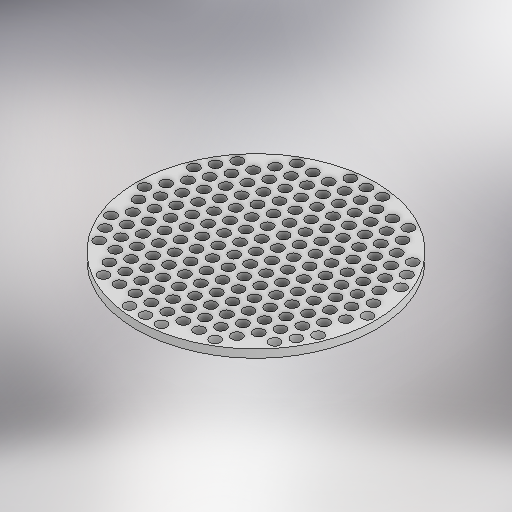
# Autodesk Inventor part: 滤网
Saved by Autodesk Inventor 2025 (Build 290162000, 162)
## iProperties
Created: 2025-03-16
Part Number: 滤网
Material: 常规
Document SubType Name: Modeling
Designer: ASUS
Density: 1 g/cm^3
Appearance: 默认
Author: ASUS
Autodesk Inventor part; units mm, degrees
ref_plane "YZ Plane" through (0, 0, 0) normal (1, 0, 0) x (0, 1, 0)
ref_plane "XZ Plane" through (0, 0, 0) normal (0, 1, 0) x (-1, 0, 0)
ref_plane "XY Plane" through (0, 0, 0) normal (0, 0, 1) x (1, 0, 0)
sketch "草图2" plane through (0, 0, 0) normal (0, 1, 0) x (1, 0, 0)
  circle A0 centre (0, 0) radius 1
  circle A1 centre (-1.5, -2.5981) radius 1
  circle A2 centre (1.5, -2.5981) radius 1
  circle A3 centre (-3, -20.7846) radius 1
  circle A4 centre (0, -20.7846) radius 1
  circle A5 centre (3, -20.7846) radius 1
  circle A6 centre (7.5, -18.1865) radius 1
  circle A7 centre (4.5, -18.1865) radius 1
  circle A8 centre (1.5, -18.1865) radius 1
  circle A9 centre (-1.5, -18.1865) radius 1
  circle A10 centre (-4.5, -18.1865) radius 1
  circle A11 centre (-7.5, -18.1865) radius 1
  circle A12 centre (-10.5, -18.1865) radius 1
  circle A13 centre (10.5, -18.1865) radius 1
  circle A14 centre (12, -15.5885) radius 1
  circle A15 centre (9, -15.5885) radius 1
  circle A16 centre (6, -15.5885) radius 1
  circle A17 centre (3, -15.5885) radius 1
  circle A18 centre (0, -15.5885) radius 1
  circle A19 centre (-3, -15.5885) radius 1
  circle A20 centre (-6, -15.5885) radius 1
  circle A21 centre (-9, -15.5885) radius 1
  circle A22 centre (-16.5, -12.9904) radius 1
  circle A23 centre (-13.5, -12.9904) radius 1
  circle A24 centre (-10.5, -12.9904) radius 1
  circle A25 centre (-7.5, -12.9904) radius 1
  circle A26 centre (-4.5, -12.9904) radius 1
  circle A27 centre (-1.5, -12.9904) radius 1
  circle A28 centre (1.5, -12.9904) radius 1
  circle A29 centre (4.5, -12.9904) radius 1
  circle A30 centre (7.5, -12.9904) radius 1
  circle A31 centre (10.5, -12.9904) radius 1
  circle A32 centre (13.5, -12.9904) radius 1
  circle A33 centre (16.5, -12.9904) radius 1
  circle A34 centre (18, -10.3923) radius 1
  circle A35 centre (15, -10.3923) radius 1
  circle A36 centre (12, -10.3923) radius 1
  circle A37 centre (9, -10.3923) radius 1
  circle A38 centre (6, -10.3923) radius 1
  circle A39 centre (3, -10.3923) radius 1
  circle A40 centre (0, -10.3923) radius 1
  circle A41 centre (-3, -10.3923) radius 1
  circle A42 centre (-6, -10.3923) radius 1
  circle A43 centre (-9, -10.3923) radius 1
  circle A44 centre (-12, -10.3923) radius 1
  circle A45 centre (-15, -10.3923) radius 1
  circle A46 centre (-18, -10.3923) radius 1
  circle A47 centre (-16.5, -7.7942) radius 1
  circle A48 centre (-13.5, -7.7942) radius 1
  circle A49 centre (-15, -5.1962) radius 1
  circle A50 centre (-18, -5.1962) radius 1
  circle A51 centre (-10.5, -7.7942) radius 1
  circle A52 centre (-7.5, -7.7942) radius 1
  circle A53 centre (-12, -5.1962) radius 1
  circle A54 centre (-6, -5.1962) radius 1
  circle A55 centre (-3, -5.1962) radius 1
  circle A56 centre (-4.5, -7.7942) radius 1
  circle A57 centre (-1.5, -7.7942) radius 1
  circle A58 centre (0, -5.1962) radius 1
  circle A59 centre (3, -5.1962) radius 1
  circle A60 centre (1.5, -7.7942) radius 1
  circle A61 centre (4.5, -7.7942) radius 1
  circle A62 centre (6, -5.1962) radius 1
  circle A63 centre (9, -5.1962) radius 1
  circle A64 centre (7.5, -7.7942) radius 1
  circle A65 centre (10.5, -7.7942) radius 1
  circle A66 centre (13.5, -7.7942) radius 1
  circle A67 centre (12, -5.1962) radius 1
  circle A68 centre (15, -5.1962) radius 1
  circle A69 centre (18, -5.1962) radius 1
  circle A70 centre (19.5, -7.7942) radius 1
  circle A71 centre (16.5, -7.7942) radius 1
  circle A72 centre (-12, -15.5885) radius 1
  circle A73 centre (-9, -5.1962) radius 1
  circle A74 centre (-19.5, -7.7942) radius 1
  circle A75 centre (-19.5, -2.5981) radius 1
  circle A76 centre (-16.5, -2.5981) radius 1
  circle A77 centre (-13.5, -2.5981) radius 1
  circle A78 centre (-10.5, -2.5981) radius 1
  circle A79 centre (-7.5, -2.5981) radius 1
  circle A80 centre (-4.5, -2.5981) radius 1
  circle A81 centre (4.5, -2.5981) radius 1
  circle A82 centre (7.5, -2.5981) radius 1
  circle A83 centre (10.5, -2.5981) radius 1
  circle A84 centre (13.5, -2.5981) radius 1
  circle A85 centre (16.5, -2.5981) radius 1
  circle A86 centre (19.5, -2.5981) radius 1
  line L0 (-23.4041, 0) -> (24.2926, 0) construction
  circle A87 centre (-1.5, 2.5981) radius 1
  circle A88 centre (1.5, 2.5981) radius 1
  circle A89 centre (-3, 20.7846) radius 1
  circle A90 centre (0, 20.7846) radius 1
  circle A91 centre (3, 20.7846) radius 1
  circle A92 centre (7.5, 18.1865) radius 1
  circle A93 centre (4.5, 18.1865) radius 1
  circle A94 centre (1.5, 18.1865) radius 1
  circle A95 centre (-1.5, 18.1865) radius 1
  circle A96 centre (-4.5, 18.1865) radius 1
  circle A97 centre (-7.5, 18.1865) radius 1
  circle A98 centre (-10.5, 18.1865) radius 1
  circle A99 centre (10.5, 18.1865) radius 1
  circle A100 centre (12, 15.5885) radius 1
  circle A101 centre (9, 15.5885) radius 1
  circle A102 centre (6, 15.5885) radius 1
  circle A103 centre (3, 15.5885) radius 1
  circle A104 centre (0, 15.5885) radius 1
  circle A105 centre (-3, 15.5885) radius 1
  circle A106 centre (-6, 15.5885) radius 1
  circle A107 centre (-9, 15.5885) radius 1
  circle A108 centre (-16.5, 12.9904) radius 1
  circle A109 centre (-13.5, 12.9904) radius 1
  circle A110 centre (-10.5, 12.9904) radius 1
  circle A111 centre (-7.5, 12.9904) radius 1
  circle A112 centre (-4.5, 12.9904) radius 1
  circle A113 centre (-1.5, 12.9904) radius 1
  circle A114 centre (1.5, 12.9904) radius 1
  circle A115 centre (4.5, 12.9904) radius 1
  circle A116 centre (7.5, 12.9904) radius 1
  circle A117 centre (10.5, 12.9904) radius 1
  circle A118 centre (13.5, 12.9904) radius 1
  circle A119 centre (16.5, 12.9904) radius 1
  circle A120 centre (18, 10.3923) radius 1
  circle A121 centre (15, 10.3923) radius 1
  circle A122 centre (12, 10.3923) radius 1
  circle A123 centre (9, 10.3923) radius 1
  circle A124 centre (6, 10.3923) radius 1
  circle A125 centre (3, 10.3923) radius 1
  circle A126 centre (0, 10.3923) radius 1
  circle A127 centre (-3, 10.3923) radius 1
  circle A128 centre (-6, 10.3923) radius 1
  circle A129 centre (-9, 10.3923) radius 1
  circle A130 centre (-12, 10.3923) radius 1
  circle A131 centre (-15, 10.3923) radius 1
  circle A132 centre (-18, 10.3923) radius 1
  circle A133 centre (-16.5, 7.7942) radius 1
  circle A134 centre (-13.5, 7.7942) radius 1
  circle A135 centre (-15, 5.1962) radius 1
  circle A136 centre (-18, 5.1962) radius 1
  circle A137 centre (-10.5, 7.7942) radius 1
  circle A138 centre (-7.5, 7.7942) radius 1
  circle A139 centre (-12, 5.1962) radius 1
  circle A140 centre (-6, 5.1962) radius 1
  circle A141 centre (-3, 5.1962) radius 1
  circle A142 centre (-4.5, 7.7942) radius 1
  circle A143 centre (-1.5, 7.7942) radius 1
  circle A144 centre (0, 5.1962) radius 1
  circle A145 centre (3, 5.1962) radius 1
  circle A146 centre (1.5, 7.7942) radius 1
  circle A147 centre (4.5, 7.7942) radius 1
  circle A148 centre (6, 5.1962) radius 1
  circle A149 centre (9, 5.1962) radius 1
  circle A150 centre (7.5, 7.7942) radius 1
  circle A151 centre (10.5, 7.7942) radius 1
  circle A152 centre (13.5, 7.7942) radius 1
  circle A153 centre (12, 5.1962) radius 1
  circle A154 centre (15, 5.1962) radius 1
  circle A155 centre (18, 5.1962) radius 1
  circle A156 centre (19.5, 7.7942) radius 1
  circle A157 centre (16.5, 7.7942) radius 1
  circle A158 centre (-12, 15.5885) radius 1
  circle A159 centre (-9, 5.1962) radius 1
  circle A160 centre (-19.5, 7.7942) radius 1
  circle A161 centre (-19.5, 2.5981) radius 1
  circle A162 centre (-16.5, 2.5981) radius 1
  circle A163 centre (-13.5, 2.5981) radius 1
  circle A164 centre (-10.5, 2.5981) radius 1
  circle A165 centre (-7.5, 2.5981) radius 1
  circle A166 centre (-4.5, 2.5981) radius 1
  circle A167 centre (4.5, 2.5981) radius 1
  circle A168 centre (7.5, 2.5981) radius 1
  circle A169 centre (10.5, 2.5981) radius 1
  circle A170 centre (13.5, 2.5981) radius 1
  circle A171 centre (16.5, 2.5981) radius 1
  circle A172 centre (19.5, 2.5981) radius 1
  circle A173 centre (-3, 0) radius 1
  circle A174 centre (-6, 0) radius 1
  circle A175 centre (-9, 0) radius 1
  circle A176 centre (-12, 0) radius 1
  circle A177 centre (-15, 0) radius 1
  circle A178 centre (-18, 0) radius 1
  circle A179 centre (-21, 0) radius 1
  circle A180 centre (3, 0) radius 1
  circle A181 centre (6, 0) radius 1
  circle A182 centre (9, 0) radius 1
  circle A183 centre (12, 0) radius 1
  circle A184 centre (15, 0) radius 1
  circle A185 centre (18, 0) radius 1
  circle A186 centre (21, 0) radius 1
  circle A187 centre (0, 0) radius 22.5
  dimension "d27" = 2
  dimension "d28" = 2
  dimension "d29" = 2
  dimension "d30" = 2
  dimension "d31" = 2
  dimension "d32" = 2
  dimension "d33" = 2
  dimension "d34" = 2
  dimension "d35" = 2
  dimension "d36" = 2
  dimension "d37" = 2
  dimension "d38" = 2
  dimension "d39" = 2
  dimension "d42" = 2
  dimension "d44" = 2
  dimension "d45" = 2
  dimension "d46" = 2
  dimension "d47" = 2
  dimension "d48" = 2
  dimension "d49" = 2
  dimension "d50" = 2
  dimension "d51" = 2
  dimension "d55" = 2
  dimension "d56" = 2
  dimension "d57" = 2
  dimension "d58" = 2
  dimension "d59" = 2
  dimension "d60" = 2
  dimension "d61" = 2
  dimension "d62" = 2
  dimension "d63" = 2
  dimension "d64" = 2
  dimension "d65" = 2
  dimension "d66" = 2
  dimension "d67" = 2
  dimension "d68" = 2
  dimension "d69" = 2
  dimension "d70" = 2
  dimension "d71" = 2
  dimension "d72" = 2
  dimension "d73" = 2
  dimension "d74" = 2
  dimension "d75" = 2
  dimension "d76" = 2
  dimension "d77" = 2
  dimension "d78" = 2
  dimension "d79" = 2
  dimension "d82" = 2
  dimension "d83" = 2
  dimension "d84" = 2
  dimension "d85" = 2
  dimension "d86" = 2
  dimension "d87" = 2
  dimension "d89" = 2
  dimension "d91" = 2
  dimension "d92" = 2
  dimension "d94" = 2
  dimension "d95" = 2
  dimension "d96" = 2
  dimension "d97" = 2
  dimension "d98" = 2
  dimension "d99" = 2
  dimension "d100" = 2
  dimension "d101" = 2
  constraints: 188 centre point, 172 symmetric about line, 2 coincident, 2 end point, 1 horizontal, 86 other
  measures "d27" diameter of A0
  measures "d28" diameter of A1
  measures "d29" diameter of A2
  measures "d30" diameter of A3
  measures "d31" diameter of A4
  measures "d32" diameter of A5
  measures "d33" diameter of A6
  measures "d34" diameter of A7
  measures "d35" diameter of A8
  measures "d36" diameter of A9
  measures "d37" diameter of A10
  measures "d38" diameter of A11
  measures "d39" diameter of A12
  measures "d42" diameter of A13
  measures "d44" diameter of A14
  measures "d45" diameter of A15
  measures "d46" diameter of A16
  measures "d47" diameter of A17
  measures "d48" diameter of A18
  measures "d49" diameter of A19
  measures "d50" diameter of A20
  measures "d51" diameter of A21
  measures "d55" diameter of A22
  measures "d56" diameter of A23
  measures "d57" diameter of A24
  measures "d58" diameter of A25
  measures "d59" diameter of A26
  measures "d60" diameter of A27
  measures "d61" diameter of A28
  measures "d62" diameter of A29
  measures "d63" diameter of A30
  measures "d64" diameter of A31
  measures "d65" diameter of A32
  measures "d66" diameter of A33
  measures "d67" diameter of A34
  measures "d68" diameter of A35
  measures "d69" diameter of A36
  measures "d70" diameter of A37
  measures "d71" diameter of A38
  measures "d72" diameter of A39
  measures "d73" diameter of A40
  measures "d74" diameter of A41
  measures "d75" diameter of A42
  measures "d76" diameter of A43
  measures "d77" diameter of A44
  measures "d78" diameter of A45
  measures "d79" diameter of A46
  measures "d82" diameter of A47
  measures "d83" diameter of A48
  measures "d84" diameter of A49
  measures "d85" diameter of A50
  measures "d86" diameter of A51
  measures "d87" diameter of A52
  measures "d89" diameter of A53
  measures "d91" diameter of A54
  measures "d92" diameter of A55
  measures "d94" diameter of A56
  measures "d95" diameter of A57
  measures "d96" diameter of A58
  measures "d97" diameter of A59
  measures "d98" diameter of A60
  measures "d99" diameter of A61
  measures "d100" diameter of A62
  measures "d101" diameter of A63
extrude "拉伸2" add sketch "草图2" against normal blind 1.5
